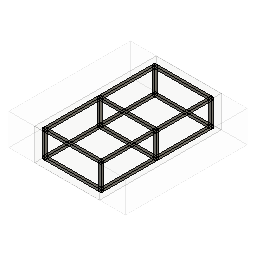
GP_TARS_V2_1000_NARROW480_CAGE_V1 (Autodesk Fusion 360 design; units mm, degrees)
part number: 2026-08-09-22-17-13-178
part number: 2026-08-09-22-17-13-287
part number: 2026-08-09-22-17-13-365
part number: 2026-08-09-22-17-13-377
part number: 2026-08-09-22-17-13-401
part number: 2026-08-09-22-17-13-418
part number: 2026-08-09-22-17-13-434
part number: 2026-08-09-22-17-13-451
part number: 2026-08-09-22-17-13-469
part number: 2026-08-09-22-17-13-489
part number: 2026-08-09-22-17-13-507
part number: 2026-08-09-22-17-13-528
part number: 2026-08-09-22-17-13-550
part number: 2026-08-09-22-17-13-571
part number: 2026-08-09-22-17-13-592
part number: 2026-08-09-22-17-59-087
part number: 2026-08-09-22-17-59-122
part number: 2026-08-09-22-17-59-149
part number: 2026-08-09-22-17-59-176
Autodesk Fusion 360 part; units mm, degrees
sketch "Overall_Envelope_1m_Profile" plane through (0, 0, 0) normal (0, 0, 1) x (1, 0, 0) in component "Overall_Envelope_1m"
  line L0 (-479.3589, 0) -> (479.3589, 0)
  line L1 (479.3589, 0) -> (479.3589, 1000)
  line L2 (479.3589, 1000) -> (-479.3589, 1000)
  line L3 (-479.3589, 1000) -> (-479.3589, 0)
extrude "Extrude1" add sketch "Overall_Envelope_1m_Profile" along normal blind 259.8674 makes body 1 in component "Overall_Envelope_1m"
sketch "Central_Chassis_Envelope_Profile" plane through (0, 0, 0) normal (0, 0, 1) x (1, 0, 0) in component "Central_Chassis_Envelope"
  line L0 (-266.0414, 0) -> (266.0414, 0)
  line L1 (266.0414, 0) -> (266.0414, 998.6144)
  line L2 (266.0414, 998.6144) -> (-266.0414, 998.6144)
  line L3 (-266.0414, 998.6144) -> (-266.0414, 0)
extrude "Extrude1'" add sketch "Central_Chassis_Envelope_Profile" along normal blind 259.8674 separate body makes body 2 in component "Central_Chassis_Envelope"
sketch "Frame_Vert_LF_Profile" plane through (0, 0, 0) normal (0, 0, 1) x (1, 0, 0) in component "Frame_Vert_LF"
  line L0 (-241.0414, 40) -> (-221.0414, 40)
  line L1 (-221.0414, 40) -> (-221.0414, 960)
  line L2 (-221.0414, 960) -> (-241.0414, 960)
  line L3 (-241.0414, 960) -> (-241.0414, 40)
extrude "Extrude1''" add sketch "Frame_Vert_LF_Profile" along normal blind 20 separate body makes body 3 in component "Frame_Vert_LF"
move_body "Move1" bodies 3 to x (1, 0, 0) y (0, 1, 0) z (0, 0, 1) at (0, 0, 20) in component "Frame_Vert_LF"
sketch "Frame_Vert_LB_Profile" plane through (0, 0, 0) normal (0, 0, 1) x (1, 0, 0) in component "Frame_Vert_LB"
  line L0 (-241.0414, 40) -> (-221.0414, 40)
  line L1 (-221.0414, 40) -> (-221.0414, 960)
  line L2 (-221.0414, 960) -> (-241.0414, 960)
  line L3 (-241.0414, 960) -> (-241.0414, 40)
extrude "Extrude1'''" add sketch "Frame_Vert_LB_Profile" along normal blind 20 separate body makes body 4 in component "Frame_Vert_LB"
move_body "Move1'" bodies 4 to x (1, 0, 0) y (0, 1, 0) z (0, 0, 1) at (0, 0, 219.8674) in component "Frame_Vert_LB"
sketch "Frame_Vert_RF_Profile" plane through (0, 0, 0) normal (0, 0, 1) x (1, 0, 0) in component "Frame_Vert_RF"
  line L0 (221.0414, 40) -> (241.0414, 40)
  line L1 (241.0414, 40) -> (241.0414, 960)
  line L2 (241.0414, 960) -> (221.0414, 960)
  line L3 (221.0414, 960) -> (221.0414, 40)
extrude "Extrude1''''" add sketch "Frame_Vert_RF_Profile" along normal blind 20 separate body makes body 5 in component "Frame_Vert_RF"
move_body "Move1''" bodies 5 to x (1, 0, 0) y (0, 1, 0) z (0, 0, 1) at (0, 0, 20) in component "Frame_Vert_RF"
sketch "Frame_Vert_RB_Profile" plane through (0, 0, 0) normal (0, 0, 1) x (1, 0, 0) in component "Frame_Vert_RB"
  line L0 (221.0414, 40) -> (241.0414, 40)
  line L1 (241.0414, 40) -> (241.0414, 960)
  line L2 (241.0414, 960) -> (221.0414, 960)
  line L3 (221.0414, 960) -> (221.0414, 40)
extrude "Extrude1'''''" add sketch "Frame_Vert_RB_Profile" along normal blind 20 separate body makes body 6 in component "Frame_Vert_RB"
move_body "Move1'''" bodies 6 to x (1, 0, 0) y (0, 1, 0) z (0, 0, 1) at (0, 0, 219.8674) in component "Frame_Vert_RB"
sketch "Frame_Cross_Bottom_F_Profile" plane through (0, 0, 0) normal (0, 0, 1) x (1, 0, 0) in component "Frame_Cross_Bottom_F"
  line L0 (-241.0414, 40) -> (241.0414, 40)
  line L1 (241.0414, 40) -> (241.0414, 60)
  line L2 (241.0414, 60) -> (-241.0414, 60)
  line L3 (-241.0414, 60) -> (-241.0414, 40)
extrude "Extrude1''''''" add sketch "Frame_Cross_Bottom_F_Profile" along normal blind 20 separate body makes body 7 in component "Frame_Cross_Bottom_F"
move_body "Move1''''" bodies 7 to x (1, 0, 0) y (0, 1, 0) z (0, 0, 1) at (0, 0, 20) in component "Frame_Cross_Bottom_F"
sketch "Frame_Cross_Bottom_B_Profile" plane through (0, 0, 0) normal (0, 0, 1) x (1, 0, 0) in component "Frame_Cross_Bottom_B"
  line L0 (-241.0414, 40) -> (241.0414, 40)
  line L1 (241.0414, 40) -> (241.0414, 60)
  line L2 (241.0414, 60) -> (-241.0414, 60)
  line L3 (-241.0414, 60) -> (-241.0414, 40)
extrude "Extrude1'''''''" add sketch "Frame_Cross_Bottom_B_Profile" along normal blind 20 separate body makes body 8 in component "Frame_Cross_Bottom_B"
move_body "Move1'''''" bodies 8 to x (1, 0, 0) y (0, 1, 0) z (0, 0, 1) at (0, 0, 219.8674) in component "Frame_Cross_Bottom_B"
sketch "Frame_Cross_Top_F_Profile" plane through (0, 0, 0) normal (0, 0, 1) x (1, 0, 0) in component "Frame_Cross_Top_F"
  line L0 (-241.0414, 940) -> (241.0414, 940)
  line L1 (241.0414, 940) -> (241.0414, 960)
  line L2 (241.0414, 960) -> (-241.0414, 960)
  line L3 (-241.0414, 960) -> (-241.0414, 940)
extrude "Extrude1''''''''" add sketch "Frame_Cross_Top_F_Profile" along normal blind 20 separate body makes body 9 in component "Frame_Cross_Top_F"
move_body "Move1''''''" bodies 9 to x (1, 0, 0) y (0, 1, 0) z (0, 0, 1) at (0, 0, 20) in component "Frame_Cross_Top_F"
sketch "Frame_Cross_Top_B_Profile" plane through (0, 0, 0) normal (0, 0, 1) x (1, 0, 0) in component "Frame_Cross_Top_B"
  line L0 (-241.0414, 940) -> (241.0414, 940)
  line L1 (241.0414, 940) -> (241.0414, 960)
  line L2 (241.0414, 960) -> (-241.0414, 960)
  line L3 (-241.0414, 960) -> (-241.0414, 940)
extrude "Extrude1'''''''''" add sketch "Frame_Cross_Top_B_Profile" along normal blind 20 separate body makes body 10 in component "Frame_Cross_Top_B"
move_body "Move1'''''''" bodies 10 to x (1, 0, 0) y (0, 1, 0) z (0, 0, 1) at (0, 0, 219.8674) in component "Frame_Cross_Top_B"
sketch "Frame_Depth_Bottom_L_Profile" plane through (0, 0, 0) normal (0, 0, 1) x (1, 0, 0) in component "Frame_Depth_Bottom_L"
  line L0 (-241.0414, 40) -> (-221.0414, 40)
  line L1 (-221.0414, 40) -> (-221.0414, 60)
  line L2 (-221.0414, 60) -> (-241.0414, 60)
  line L3 (-241.0414, 60) -> (-241.0414, 40)
extrude "Extrude1''''''''''" add sketch "Frame_Depth_Bottom_L_Profile" along normal blind 219.8674 separate body makes body 11 in component "Frame_Depth_Bottom_L"
move_body "Move1''''''''" bodies 11 to x (1, 0, 0) y (0, 1, 0) z (0, 0, 1) at (0, 0, 20) in component "Frame_Depth_Bottom_L"
sketch "Frame_Depth_Bottom_R_Profile" plane through (0, 0, 0) normal (0, 0, 1) x (1, 0, 0) in component "Frame_Depth_Bottom_R"
  line L0 (221.0414, 40) -> (241.0414, 40)
  line L1 (241.0414, 40) -> (241.0414, 60)
  line L2 (241.0414, 60) -> (221.0414, 60)
  line L3 (221.0414, 60) -> (221.0414, 40)
extrude "Extrude1'''''''''''" add sketch "Frame_Depth_Bottom_R_Profile" along normal blind 219.8674 separate body makes body 12 in component "Frame_Depth_Bottom_R"
move_body "Move1'''''''''" bodies 12 to x (1, 0, 0) y (0, 1, 0) z (0, 0, 1) at (0, 0, 20) in component "Frame_Depth_Bottom_R"
sketch "Frame_Depth_Top_L_Profile" plane through (0, 0, 0) normal (0, 0, 1) x (1, 0, 0) in component "Frame_Depth_Top_L"
  line L0 (-241.0414, 940) -> (-221.0414, 940)
  line L1 (-221.0414, 940) -> (-221.0414, 960)
  line L2 (-221.0414, 960) -> (-241.0414, 960)
  line L3 (-241.0414, 960) -> (-241.0414, 940)
extrude "Extrude1''''''''''''" add sketch "Frame_Depth_Top_L_Profile" along normal blind 219.8674 separate body makes body 13 in component "Frame_Depth_Top_L"
move_body "Move1''''''''''" bodies 13 to x (1, 0, 0) y (0, 1, 0) z (0, 0, 1) at (0, 0, 20) in component "Frame_Depth_Top_L"
sketch "Frame_Depth_Top_R_Profile" plane through (0, 0, 0) normal (0, 0, 1) x (1, 0, 0) in component "Frame_Depth_Top_R"
  line L0 (221.0414, 940) -> (241.0414, 940)
  line L1 (241.0414, 940) -> (241.0414, 960)
  line L2 (241.0414, 960) -> (221.0414, 960)
  line L3 (221.0414, 960) -> (221.0414, 940)
extrude "Extrude1'''''''''''''" add sketch "Frame_Depth_Top_R_Profile" along normal blind 219.8674 separate body makes body 14 in component "Frame_Depth_Top_R"
move_body "Move1'''''''''''" bodies 14 to x (1, 0, 0) y (0, 1, 0) z (0, 0, 1) at (0, 0, 20) in component "Frame_Depth_Top_R"
sketch "Frame_Cross_Mid_F_Profile" plane through (0, 0, 0) normal (0, 0, 1) x (1, 0, 0) in component "Frame_Cross_Mid_F"
  line L0 (-241.0414, 490) -> (241.0414, 490)
  line L1 (241.0414, 490) -> (241.0414, 510)
  line L2 (241.0414, 510) -> (-241.0414, 510)
  line L3 (-241.0414, 510) -> (-241.0414, 490)
extrude "Extrude1''''''''''''''" add sketch "Frame_Cross_Mid_F_Profile" along normal blind 20 separate body makes body 15 in component "Frame_Cross_Mid_F"
move_body "Move1''''''''''''" bodies 15 to x (1, 0, 0) y (0, 1, 0) z (0, 0, 1) at (0, 0, 20) in component "Frame_Cross_Mid_F"
sketch "Frame_Cross_Mid_B_Profile" plane through (0, 0, 0) normal (0, 0, 1) x (1, 0, 0) in component "Frame_Cross_Mid_B"
  line L0 (-241.0414, 490) -> (241.0414, 490)
  line L1 (241.0414, 490) -> (241.0414, 510)
  line L2 (241.0414, 510) -> (-241.0414, 510)
  line L3 (-241.0414, 510) -> (-241.0414, 490)
extrude "Extrude1'''''''''''''''" add sketch "Frame_Cross_Mid_B_Profile" along normal blind 20 separate body makes body 16 in component "Frame_Cross_Mid_B"
move_body "Move1'''''''''''''" bodies 16 to x (1, 0, 0) y (0, 1, 0) z (0, 0, 1) at (0, 0, 219.8674) in component "Frame_Cross_Mid_B"
sketch "Frame_Depth_Mid_L_Profile" plane through (0, 0, 0) normal (0, 0, 1) x (1, 0, 0) in component "Frame_Depth_Mid_L"
  line L0 (-241.0414, 490) -> (-221.0414, 490)
  line L1 (-221.0414, 490) -> (-221.0414, 510)
  line L2 (-221.0414, 510) -> (-241.0414, 510)
  line L3 (-241.0414, 510) -> (-241.0414, 490)
extrude "Extrude1''''''''''''''''" add sketch "Frame_Depth_Mid_L_Profile" along normal blind 219.8674 separate body makes body 17 in component "Frame_Depth_Mid_L"
move_body "Move1''''''''''''''" bodies 17 to x (1, 0, 0) y (0, 1, 0) z (0, 0, 1) at (0, 0, 20) in component "Frame_Depth_Mid_L"
sketch "Frame_Depth_Mid_R_Profile" plane through (0, 0, 0) normal (0, 0, 1) x (1, 0, 0) in component "Frame_Depth_Mid_R"
  line L0 (221.0414, 490) -> (241.0414, 490)
  line L1 (241.0414, 490) -> (241.0414, 510)
  line L2 (241.0414, 510) -> (221.0414, 510)
  line L3 (221.0414, 510) -> (221.0414, 490)
extrude "Extrude1'''''''''''''''''" add sketch "Frame_Depth_Mid_R_Profile" along normal blind 219.8674 separate body makes body 18 in component "Frame_Depth_Mid_R"
move_body "Move1'''''''''''''''" bodies 18 to x (1, 0, 0) y (0, 1, 0) z (0, 0, 1) at (0, 0, 20) in component "Frame_Depth_Mid_R"
component "Overall_Envelope_1m" placed x (1, 0, 0) y (0, 1, 0) z (0, 0, 1) at (0, 0, 0)
component "Central_Chassis_Envelope" placed x (1, 0, 0) y (0, 1, 0) z (0, 0, 1) at (0, 0, 0)
component "Frame_Vert_LF" placed x (1, 0, 0) y (0, 1, 0) z (0, 0, 1) at (0, 0, 0)
component "Frame_Vert_LB" placed x (1, 0, 0) y (0, 1, 0) z (0, 0, 1) at (0, 0, 0)
component "Frame_Vert_RF" placed x (1, 0, 0) y (0, 1, 0) z (0, 0, 1) at (0, 0, 0)
component "Frame_Vert_RB" placed x (1, 0, 0) y (0, 1, 0) z (0, 0, 1) at (0, 0, 0)
component "Frame_Cross_Bottom_F" placed x (1, 0, 0) y (0, 1, 0) z (0, 0, 1) at (0, 0, 0)
component "Frame_Cross_Bottom_B" placed x (1, 0, 0) y (0, 1, 0) z (0, 0, 1) at (0, 0, 0)
component "Frame_Cross_Top_F" placed x (1, 0, 0) y (0, 1, 0) z (0, 0, 1) at (0, 0, 0)
component "Frame_Cross_Top_B" placed x (1, 0, 0) y (0, 1, 0) z (0, 0, 1) at (0, 0, 0)
component "Frame_Depth_Bottom_L" placed x (1, 0, 0) y (0, 1, 0) z (0, 0, 1) at (0, 0, 0)
component "Frame_Depth_Bottom_R" placed x (1, 0, 0) y (0, 1, 0) z (0, 0, 1) at (0, 0, 0)
component "Frame_Depth_Top_L" placed x (1, 0, 0) y (0, 1, 0) z (0, 0, 1) at (0, 0, 0)
component "Frame_Depth_Top_R" placed x (1, 0, 0) y (0, 1, 0) z (0, 0, 1) at (0, 0, 0)
component "Frame_Cross_Mid_F" placed x (1, 0, 0) y (0, 1, 0) z (0, 0, 1) at (0, 0, 0)
component "Frame_Cross_Mid_B" placed x (1, 0, 0) y (0, 1, 0) z (0, 0, 1) at (0, 0, 0)
component "Frame_Depth_Mid_L" placed x (1, 0, 0) y (0, 1, 0) z (0, 0, 1) at (0, 0, 0)
component "Frame_Depth_Mid_R" placed x (1, 0, 0) y (0, 1, 0) z (0, 0, 1) at (0, 0, 0)
equation "TARS_Height = 1000 mm" comment "Overall target height"
equation "TARS_Width = 958.717706 mm" comment "Scaled reference width"
equation "TARS_Depth = 259.867417 mm" comment "Scaled reference depth"
equation "Chassis_Width = 532.082896 mm" comment "Scaled central chassis width"
equation "Frame_Profile = 20 mm" comment "Aluminium extrusion profile"
equation "Frame_Side_Inset = 35 mm" comment "Frame inset from chassis sides"
equation "Frame_End_Inset = 40 mm" comment "Frame inset from top and bottom"
equation "Frame_Depth_Inset = 20 mm" comment "Frame inset from front and rear"
named bodies: "Overall_Envelope_1m", "Central_Chassis_Envelope", "Frame_Vert_LF", "Frame_Vert_LB", "Frame_Vert_RF", "Frame_Vert_RB", "Frame_Cross_Bottom_F", "Frame_Cross_Bottom_B", "Frame_Cross_Top_F", "Frame_Cross_Top_B", "Frame_Depth_Bottom_L", "Frame_Depth_Bottom_R", "Frame_Depth_Top_L", "Frame_Depth_Top_R", "Frame_Cross_Mid_F", "Frame_Cross_Mid_B", "Frame_Depth_Mid_L", "Frame_Depth_Mid_R"
